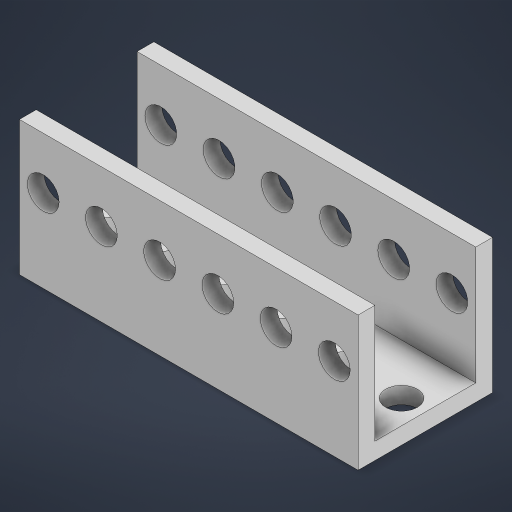
# Autodesk Inventor part: ArmSupport_C-Channel
Saved by Autodesk Inventor 2024 (Build 280153000, 153)
## iProperties
Created: 2023-11-24
Part Number: ArmSupport_C-Channel
Material: Generic
Document SubType Name: Modeling
Designer: avsar
Density: 1 g/cm^3
Appearance: Default
Author: avsar
Autodesk Inventor part; units mm, degrees
ref_plane "YZ Plane" through (0, 0, 0) normal (1, 0, 0) x (0, 1, 0)
ref_plane "XZ Plane" through (0, 0, 0) normal (0, 1, 0) x (-1, 0, 0)
ref_plane "XY Plane" through (0, 0, 0) normal (0, 0, 1) x (1, 0, 0)
sketch "Sketch1" plane through (0, 0, 0) normal (1, 0, 0) x (0, 1, 0)
  line L0 (0, 12.7) -> (0, -12.7)
  line L1 (0, 12.7) -> (25.4, 12.7)
  line L2 (0, -12.7) -> (25.4, -12.7)
  line L3 (25.4, 9.525) -> (3.175, 9.525)
  line L4 (3.175, 9.525) -> (3.175, -9.525)
  line L5 (3.175, -9.525) -> (25.4, -9.525)
  line L6 (25.4, 12.7) -> (25.4, 9.525)
  line L7 (25.4, -9.525) -> (25.4, -12.7)
  point P0 (0, 0)
  point P1 (0, 0)
  dimension "d0" = 25.4
  dimension "d1" = 25.4
  dimension "d2" = 25.4
  dimension "d3" = 3.175
  constraints: 16 end point, 2 horizontal, 2 vertical, 1 coincident, 1 collinear, 1 midpoint, 2 other
  measures "d0" distance of L0.start L0.end
  measures "d1" distance of L0.start L1.end
  measures "d2" distance of L0.end L2.end
  measures "d3" distance between parallel lines of L1 L3
extrude "Extrusion1" add sketch "Sketch1" along normal mid plane 64
sketch "Sketch2" plane through (-32, 3.175, 9.525) normal (0, 1, 0) x (1, 0, 0)
  circle A0 centre (4.5, 9.525) radius 3
  line L0 (0, 0) -> (0, 19.05) construction
  line L1 (0, 19.05) -> (64, 19.05) construction
  circle A1 centre (15.5, 9.525) radius 3
  circle A2 centre (26.5, 9.525) radius 3
  circle A3 centre (37.5, 9.525) radius 3
  circle A4 centre (48.5, 9.525) radius 3
  circle A5 centre (59.5, 9.525) radius 3
  point P0 (32, 9.525)
  point P1 (0, 9.525)
  point P2 (0, 9.525)
  dimension "d6" = 6
  dimension "d7" = 4.5
  dimension "d10" = 11
  constraints: 6 centre point, 2 midpoint, 1 horizontal, 1 horizontal alignment, 10 other
  measures "d6" diameter of A0
  measures "d7" distance of point (0, 9.525) A0.centre
  measures "d10" distance of A0.centre A1.centre
extrude "Extrusion2" cut sketch "Sketch2" against normal through all
sketch "Sketch3" plane through (-32, 0, 12.7) normal (0, 0, 1) x (1, 0, 0)
  line L0 (0, 3.175) -> (64, 3.175) construction
  line L1 (64, 25.4) -> (64, 3.175) construction
  line L2 (0, 25.4) -> (64, 25.4) construction
  line L3 (0, 3.175) -> (0, 25.4) construction
  circle A0 centre (4.5, 15.625) radius 3
  circle A1 centre (15.5, 15.625) radius 3
  circle A2 centre (26.5, 15.625) radius 3
  circle A3 centre (37.5, 15.625) radius 3
  circle A4 centre (48.5, 15.625) radius 3
  circle A5 centre (59.5, 15.625) radius 3
  point P0 (32, 0)
  dimension "d17" = 6
  dimension "d18" = 12.45
  dimension "d19" = 4.5
  dimension "d22" = 11
  constraints: 6 centre point, 1 horizontal, 10 other
  measures "d17" diameter of A0
  measures "d18" distance from line of L0 A0.centre
  measures "d19" distance from line of L3 A0.centre
  measures "d22" distance of A0.centre A1.centre
extrude "Extrusion3" cut sketch "Sketch3" against normal through all
body "Solid1"
